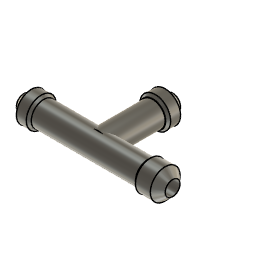
Connecteur essence en T - Petit_ (Autodesk Fusion 360 design; units mm, degrees)
Autodesk Fusion 360 part; units mm, degrees
sketch "Esquisse2" plane through (0, 0, 0) normal (1, 0, 0) x (0, 1, 0)
  circle A0 centre (0, 0) radius 1.5
  circle A1 centre (0, 0) radius 2.5
  dimension "d1" = 3
  dimension "d2" = 5
  constraint coincident A0.centre A1.centre
  measures "d1" diameter of A0
  measures "d2" diameter of A1
extrude "Extrusion1" add sketch "Esquisse2" along normal mid plane 30 makes body 1
sketch "Esquisse3" plane through (0, 0, 0) normal (0, 1, 0) x (1, 0, 0)
  circle A0 centre (0, 0) radius 1.5
  circle A1 centre (0, 0) radius 2.5
  dimension "d5" = 3
  dimension "d6" = 5
  constraint coincident A0.centre A1.centre
  measures "d5" diameter of A0
  measures "d6" diameter of A1
extrude "Extrusion2" add sketch "Esquisse3" along normal blind 15 separate body makes body 2
move_body "Déplacer1" bodies 2 1 to x (1, 0, 0) y (0, 1, 0) z (0, 0, 1) at (0, -15, 0)
sketch "Esquisse4" plane through (0, 0, 0) normal (0, 1, 0) x (-1, 0, 0)
  circle A0 centre (0, 0) radius 1.5
  circle A1 centre (0, 0) radius 2.5
  circle A2 centre (0, 0) radius 3.1
  dimension "d9" = 6.2
  constraint coincident A0.centre A1.centre
  measures "d9" diameter of A2
extrude "Extrusion3" add sketch "Esquisse4" against normal blind 4 contours A2 bodies 2
chamfer "Chanfrein1" distance 0.5 angle 45 1 edges at (2.8902, -4, 1.121) on bodies 2
chamfer "Chanfrein2" distance 1.5 angle 45 1 edges at (2.8902, 0, -1.121) on bodies 2
move_body "Déplacer2" bodies 1 2 to x (1, 0, 0) y (0, 1, 0) z (0, 0, 1) at (15, 15, 0)
sketch "Esquisse5" plane through (0, 0, 0) normal (1, 0, 0) x (0, 1, 0)
  circle A0 centre (0, 0) radius 2.5
  circle A1 centre (0, 0) radius 3
  dimension "d14" = 6
  constraint coincident A0.centre A1.centre
  measures "d14" diameter of A1
extrude "Extrusion4" add sketch "Esquisse5" along normal blind 4 bodies 1
chamfer "Chanfrein3" distance 1.5 angle 45 1 edges at (0, -2.797, -1.0848) on bodies 1
chamfer "Chanfrein4" distance 0.5 angle 45 1 edges at (4, -2.797, -1.0848) on bodies 1
move_body "Déplacer3" bodies 1 2 to x (1, 0, 0) y (0, 1, 0) z (0, 0, 1) at (-30, 0, 0)
sketch "Esquisse6" plane through (0, 0, 0) normal (1, 0, 0) x (0, 1, 0)
  circle A0 centre (0, 0) radius 1.5179
  circle A1 centre (0, 0) radius 1.5
  circle A2 centre (0, 0) radius 3
  dimension "d19" = 3
  dimension "d20" = 6
  constraint coincident A0.centre A1.centre
  constraint concentric A0 A1
  constraint concentric A0 A2
  measures "d19" diameter of A1
  measures "d20" diameter of A2
extrude "Extrusion5" add sketch "Esquisse6" against normal blind 5 contours A2 bodies 1
chamfer "Chanfrein5" distance 1.5 angle 45 1 edges at (0, -2.797, -1.0848) on bodies 1
chamfer "Chanfrein6" distance 0.5 angle 45 1 edges at (-5, -2.797, 1.0848) on bodies 1
sketch "Esquisse7" plane through (0, 0, 0) normal (1, 0, 0) x (0, 1, 0)
  circle A0 centre (0, 0) radius 1.5
  dimension "d25" = 3
  constraint coincident A0.centre origin
  measures "d25" diameter of A0
extrude "Extrusion6" cut sketch "Esquisse7" against normal blind 30 bodies 2
move_body "Déplacer4" bodies 2 1 to x (1, 0, 0) y (0, 1, 0) z (0, 0, 1) at (16, -15, 0)
move_body "Déplacer5" bodies 1 2 to x (1, 0, 0) y (0, 1, 0) z (0, 0, 1) at (-1, 0, 0)
sketch "Esquisse8" plane through (0, 0, 0) normal (0, 1, 0) x (1, 0, 0)
  circle A0 centre (0, 0) radius 1.5
  dimension "d28" = 3
  constraint coincident A0.centre origin
  measures "d28" diameter of A0
extrude "Extrusion7" cut sketch "Esquisse8" against normal blind 15.5 bodies 1
